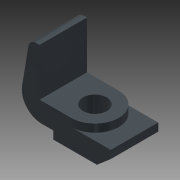
# Autodesk Inventor part: HW 4 Part 3
Saved by Autodesk Inventor 2015 SP1 (Build 190203100, 203)
## iProperties
Created: 2016-01-27
Part Number: HW 4 Part 3
Material: Iron, Cast
Document SubType Name: Modeling
Designer: melissa.roth
Density: 7.15 g/cm^3
Appearance: Iron Gray
Mass: 3206.3 g
Surface Area: 529.972 cm^2
Volume: 448.434 cm^3
Author: melissa.roth
Autodesk Inventor part; units mm, degrees
ref_plane "YZ Plane" through (0, 0, 0) normal (1, 0, 0) x (0, 1, 0)
ref_plane "XZ Plane" through (0, 0, 0) normal (0, 1, 0) x (-1, 0, 0)
ref_plane "XY Plane" through (0, 0, 0) normal (0, 0, 1) x (1, 0, 0)
sketch "Sketch1" plane through (0, 0, 0) normal (0, 0, 1) x (1, 0, 0)
  line L0 (0, 0) -> (19.05, 0)
  line L1 (19.05, 0) -> (19.05, -12.7)
  line L2 (19.05, -12.7) -> (88.9, -12.7)
  line L3 (111.125, 19.05) -> (47.625, 19.05)
  line L4 (47.625, 19.05) -> (47.625, 31.75)
  line L5 (47.625, 31.75) -> (-3.175, 31.75)
  line L6 (-3.175, 31.75) -> (-3.175, 107.95)
  line L7 (-3.175, 107.95) -> (-8.6301, 107.95)
  arc A0 (-8.6301, 107.95) -> (-21.154, 97.3579) centre (-8.6301, 95.25) ccw
  arc A1 (-31.3096, 37.0198) -> (0, 0) centre (0, 31.75) ccw
  line L8 (-31.3096, 37.0198) -> (-21.154, 97.3579)
  line L9 (88.9, -12.7) -> (111.125, 6.35)
  line L10 (111.125, 6.35) -> (111.125, 19.05)
  dimension "d29" = 114.3
  dimension "d30" = 120.65
  dimension "d31" = 19.05
  dimension "d32" = 69.85
  dimension "d33" = 50.8
  dimension "d35" = 31.75
  dimension "d36" = 76.2
  dimension "d37" = 12.7
  dimension "d38" = 31.75
  dimension "d39" = 12.7
  dimension "d40" = 12.7
  constraints: 22 end point, 5 perpendicular, 4 point on circle, 4 tangent, 2 centre point, 1 horizontal, 1 vertical
  measures "d29" horizontal distance of L3.start L6.end
  measures "d30" vertical distance of L1.end L6.end
  measures "d31" distance of L0.start L0.end
  measures "d32" distance of L1.end L2.end
  measures "d33" distance of L4.end L5.end
  measures "d35" distance between parallel lines of L0 L5
  measures "d36" distance of L5.end L6.end
  measures "d37" radius of A0
  measures "d38" radius of A1
  measures "d39" distance of L3.end L4.end
  measures "d40" distance of L9.end L3.start
extrude "Extrusion1" add sketch "Sketch1" along normal mid plane 76.2
sketch "Sketch2" plane through (47.625, 19.05, 38.1) normal (0, 1, 0) x (1, 0, 0)
  line L0 (0, 76.2) -> (0, 0) projected
  circle A0 centre (0, 38.1) radius 38.1
  point P0 (-47.625, 38.1)
  constraints: 1 midpoint, 1 vertical alignment, 2 other
extrude "Extrusion2" add sketch "Sketch2" along normal blind 12.7
hole "Hole1" at (47.625, 31.75, 0) direction (0, -1, 0) diameter 38.1 end through all
body "Solid1"
